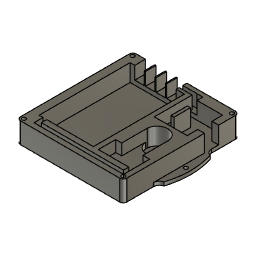
B07Z94FZSQ Wood Box v5 (Autodesk Fusion 360 design; units mm, degrees)
Autodesk Fusion 360 part; units mm, degrees
sketch "BoardDetails" plane through (0, 0, 0) normal (0, 0, 1) x (1, 0, 0)
  line L0 (6.7571, 3.9956, 17.5) -> (52.7571, 3.9956, 17.5)
  line L1 (52.7571, 3.9956, 17.5) -> (52.7571, 80.9956, 17.5)
  line L2 (52.7571, 80.9956, 17.5) -> (6.7571, 80.9956, 17.5)
  line L3 (6.7571, 80.9956, 17.5) -> (6.7571, 3.9956, 17.5)
  line L4 (29.7571, 80.9956, 17.5) -> (29.7571, 3.9956, 17.5) construction
  line L5 (29.7571, 80.9956, 17.5) -> (29.7571, 80.2494, 17.5)
  line L6 (29.7571, 80.9956, 17.5) -> (29.7571, 78.4956, 17.5) construction
  line L7 (29.7571, 78.4956, 17.5) -> (49.7571, 78.4956, 17.5) construction
  line L8 (29.7571, 78.4956, 17.5) -> (9.7571, 78.4956, 17.5) construction
  circle A0 through (12.0071, 78.4956, 17.5) (8.6321, 80.4442, 17.5) (8.6321, 76.5471, 17.5)
  circle A1 through (52.0071, 78.4956, 17.5) (48.6321, 80.4442, 17.5) (48.6321, 76.5471, 17.5)
  line L9 (29.7571, 3.9956, 17.5) -> (29.7571, 6.4956, 17.5)
  line L10 (29.7571, 6.4956, 17.5) -> (49.7571, 6.4956, 17.5) construction
  line L11 (29.7571, 6.4956, 17.5) -> (9.7571, 6.4956, 17.5) construction
  circle A2 through (12.0071, 6.4956, 17.5) (8.6321, 8.4442, 17.5) (8.6321, 4.5471, 17.5)
  circle A3 through (52.0071, 6.4956, 17.5) (48.6321, 8.4442, 17.5) (48.6321, 4.5471, 17.5)
  line L12 (62.0692, 18.5976, 17.5) -> (80.0692, 18.5976, 17.5)
  line L13 (80.0692, 18.5976, 17.5) -> (80.0692, 48.5976, 17.5)
  line L14 (80.0692, 48.5976, 17.5) -> (62.0692, 48.5976, 17.5)
  line L15 (62.0692, 48.5976, 17.5) -> (62.0692, 18.5976, 17.5)
  circle A4 through (80.095, 39.5718, 17.5) (66.5563, 47.3884, 17.5) (66.5563, 31.7552, 17.5)
  line L16 (85.7849, 18.5976, 17.5) -> (57.0002, 18.5976, 17.5)
  line L17 (57.0002, 18.5976, 17.5) -> (57.0002, 3.9337, 17.5)
  line L18 (57.0002, 3.9337, 17.5) -> (85.7849, 3.9337, 17.5)
  line L19 (85.7849, 3.9337, 17.5) -> (85.7849, 18.5976, 17.5)
  line L20 (84.3255, 51.6593, 17.5) -> (65.3255, 51.6593, 17.5)
  line L21 (65.3255, 51.6593, 17.5) -> (65.3255, 81.6593, 17.5)
  line L22 (65.3255, 81.6593, 17.5) -> (84.3255, 81.6593, 17.5)
  line L23 (84.3255, 81.6593, 17.5) -> (84.3255, 51.6593, 17.5)
  line L24 (84.3255, 66.6593, 17.5) -> (92.8255, 66.6593, 17.5)
  line L25 (92.8255, 72.6593, 17.5) -> (84.3255, 72.6593, 17.5)
  line L26 (84.3255, 72.6593, 17.5) -> (84.3255, 60.6593, 17.5)
  line L27 (84.3255, 60.6593, 17.5) -> (92.8255, 60.6593, 17.5)
  line L28 (92.8255, 60.6593, 17.5) -> (92.8255, 72.6593, 17.5)
  line L29 (92.8255, 72.6593, 17.5) -> (84.3255, 60.6593, 17.5) construction
  line L30 (84.3255, 72.6593, 17.5) -> (92.8255, 60.6593, 17.5) construction
  line L31 (65.3255, 51.6593, 17.5) -> (57.3255, 51.6593, 17.5)
  line L32 (57.3255, 51.6593, 17.5) -> (57.3255, 59.6593, 17.5)
  line L33 (57.3255, 59.6593, 17.5) -> (65.3255, 59.6593, 17.5)
  line L34 (65.3255, 59.6593, 17.5) -> (65.3255, 51.6593, 17.5)
  line L35 (65.3255, 81.6593, 17.5) -> (57.3255, 81.6593, 17.5)
  line L36 (57.3255, 81.6593, 17.5) -> (57.3255, 73.6593, 17.5)
  line L37 (57.3255, 73.6593, 17.5) -> (65.3255, 73.6593, 17.5)
  line L38 (65.3255, 73.6593, 17.5) -> (65.3255, 81.6593, 17.5)
  line L39 (85.8245, -0.5224, 17.5) -> (10.1189, -0.5224, 17.5)
  line L40 (10.1189, -0.5224, 17.5) -> (10.1189, -3.6224, 17.5)
  line L41 (10.1189, -3.6224, 17.5) -> (85.8245, -3.6224, 17.5)
  line L42 (85.8245, -3.6224, 17.5) -> (85.8245, -0.5224, 17.5)
  line L43 (10.1189, -0.5224, 17.5) -> (13.2189, -0.5224, 17.5)
  line L44 (13.2189, -0.5224, 17.5) -> (13.2189, 9.1628, 17.5)
  line L45 (13.2189, 9.1628, 17.5) -> (10.1189, 9.1628, 17.5)
  line L46 (10.1189, 9.1628, 17.5) -> (10.1189, -0.5224, 17.5)
  line L47 (85.8245, -0.5224, 17.5) -> (82.7245, -0.5224, 17.5)
  line L48 (82.7245, -0.5224, 17.5) -> (82.7245, 9.1628, 17.5)
  line L49 (82.7245, 9.1628, 17.5) -> (85.8245, 9.1628, 17.5)
  line L50 (85.8245, 9.1628, 17.5) -> (85.8245, -0.5224, 17.5)
  line L51 (6.7133, 80.7005, 17.5) -> (10.7133, 80.7005, 17.5)
  line L52 (10.7133, 80.7005, 17.5) -> (18.7133, 80.7005, 17.5)
  line L53 (18.7133, 80.7005, 17.5) -> (18.7133, 90.7005, 17.5)
  line L54 (18.7133, 90.7005, 17.5) -> (10.7133, 90.7005, 17.5)
  line L55 (10.7133, 90.7005, 17.5) -> (10.7133, 80.7005, 17.5)
  line L56 (18.7133, 80.7005, 17.5) -> (19.7133, 80.7005, 17.5)
  line L57 (19.7133, 80.7005, 17.5) -> (19.7133, 90.1133, 17.5)
  line L58 (19.7133, 90.1133, 17.5) -> (18.7133, 90.1133, 17.5)
  line L59 (18.7133, 90.1133, 17.5) -> (18.7133, 80.7005, 17.5)
  line L60 (19.7133, 80.7005, 17.5) -> (27.7133, 80.7005, 17.5)
  line L61 (27.7133, 80.7005, 17.5) -> (27.7133, 90.7005, 17.5)
  line L62 (27.7133, 90.7005, 17.5) -> (19.7133, 90.7005, 17.5)
  line L63 (19.7133, 90.7005, 17.5) -> (19.7133, 80.7005, 17.5)
  line L64 (27.7133, 80.7005, 17.5) -> (28.7133, 80.7005, 17.5)
  line L65 (28.7133, 80.7005, 17.5) -> (28.7133, 90.4026, 17.5)
  line L66 (28.7133, 90.4026, 17.5) -> (27.7133, 90.4026, 17.5)
  line L67 (27.7133, 90.4026, 17.5) -> (27.7133, 80.7005, 17.5)
  line L68 (28.7133, 80.7005, 17.5) -> (36.7133, 80.7005, 17.5)
  line L69 (36.7133, 80.7005, 17.5) -> (36.7133, 90.7005, 17.5)
  line L70 (36.7133, 90.7005, 17.5) -> (28.7133, 90.7005, 17.5)
  line L71 (28.7133, 90.7005, 17.5) -> (28.7133, 80.7005, 17.5)
  line L72 (36.7133, 80.7005, 17.5) -> (37.7133, 80.7005, 17.5)
  line L73 (37.7133, 80.7005, 17.5) -> (37.7133, 90.7005, 17.5)
  line L74 (37.7133, 90.7005, 17.5) -> (36.7133, 90.7005, 17.5)
  line L75 (36.7133, 90.7005, 17.5) -> (36.7133, 80.7005, 17.5)
  line L76 (37.7133, 80.7005, 17.5) -> (45.7133, 80.7005, 17.5)
  line L77 (45.7133, 80.7005, 17.5) -> (45.7133, 90.7005, 17.5)
  line L78 (45.7133, 90.7005, 17.5) -> (37.7133, 90.7005, 17.5)
  line L79 (37.7133, 90.7005, 17.5) -> (37.7133, 80.7005, 17.5)
  line L80 (45.7133, 83.4948, 17.5) -> (57.7133, 83.4948, 17.5)
  line L81 (57.7133, 83.4948, 17.5) -> (57.7133, 86.5948, 17.5)
  line L82 (57.7133, 86.5948, 17.5) -> (45.7133, 86.5948, 17.5)
  line L83 (45.7133, 86.5948, 17.5) -> (45.7133, 83.4948, 17.5)
  circle A5 centre (9.7649, 78.4891) radius 1
  circle A6 centre (49.8028, 78.4891) radius 1
  circle A7 centre (49.7195, 6.4968) radius 1.5
  circle A8 centre (9.7352, 6.4968) radius 1.5
  line L84 (62.7102, 86.5347, 17.5) -> (56.7102, 86.5347, 17.5)
  line L85 (56.7102, 86.5347, 17.5) -> (56.7102, 51.5347, 17.5)
  line L86 (56.7102, 51.5347, 17.5) -> (62.7102, 51.5347, 17.5)
  line L87 (62.7102, 51.5347, 17.5) -> (62.7102, 86.5347, 17.5)
  point P0 (84.3255, 66.6593)
  point P1 (88.5755, 66.6593)
  dimension "d3" = 46
  dimension "d4" = 77
  dimension "d5" = 2.5
  dimension "d6" = 20
  dimension "d7" = 20
  dimension "d8" = 4.5
  dimension "d9" = 4.5
  dimension "d10" = 2.5
  dimension "d11" = 20
  dimension "d12" = 20
  dimension "d13" = 4.5
  dimension "d14" = 4.5
  dimension "d18" = 18
  dimension "d19" = 30
  dimension "d20" = 19
  dimension "d21" = 30
  dimension "d24" = 12
  dimension "d35" = 3.1
  dimension "d36" = 3.1
  dimension "d37" = 3.1
  dimension "d40" = 4
  dimension "d41" = 8
  dimension "d42" = 10
  dimension "d43" = 1
  dimension "d44" = 8
  dimension "d45" = 10
  dimension "d46" = 1
  dimension "d47" = 8
  dimension "d48" = 10
  dimension "d49" = 1
  dimension "d50" = 10
  dimension "d51" = 8
  dimension "d52" = 10
  dimension "d53" = 12
  dimension "d54" = 3.1
  dimension "d59" = 2
  dimension "d60" = 2
  dimension "d61" = 3
  dimension "d62" = 3
  dimension "d65" = 6
  dimension "d66" = 35
  measures "d59" diameter of A5
  measures "d60" diameter of A6
  measures "d61" diameter of A7
  measures "d62" diameter of A8
sketch "WoodBoardDim" plane through (0, 0, 0) normal (0, 0, 1) x (1, 0, 0)
  line L0 (3, -8) -> (87, -8)
  line L1 (87, 90) -> (3, 90)
  line L2 (0, 17.5051) -> (0, -5)
  line L3 (0, -8) -> (0, 0)
  arc A0 (3, 90) -> (0, 87) centre (3, 87) ccw
  arc A1 (90, 87) -> (87, 90) centre (87, 87) ccw
  arc A2 (87, -8) -> (90, -5) centre (87, -5) ccw
  arc A3 (0, -5) -> (3, -8) centre (3, -5) ccw
  arc A4 (0, 17.5051) -> (-4, 22.4041) centre (-5, 17.5051) ccw
  line L4 (0, 66.4949) -> (0, 87)
  arc A5 (-4, 61.5959) -> (0, 66.4949) centre (-5, 66.4949) ccw
  line L5 (90, -5) -> (90, 17.5051)
  line L6 (90, 66.4949) -> (90, 87)
  arc A6 (90, 66.4949) -> (94, 61.5959) centre (95, 66.4949) ccw
  arc A7 (94, 22.4041) -> (90, 17.5051) centre (95, 17.5051) ccw
  line L7 (0, 66.4949) -> (0, 17.5051)
  line L8 (90, 17.5051) -> (90, 66.4949)
  circle A8 centre (3, 87) radius 1.6
  circle A9 centre (87, 87) radius 1.6
  circle A10 centre (3, -5) radius 1.6
  circle A11 centre (87, -5) radius 1.6
  circle A12 centre (-3, 42) radius 1.6
  circle A13 centre (93, 42) radius 1.6
  line L9 (-3, 42) -> (-7, 42)
  line L10 (93, 42) -> (97, 42)
  spline S0 degree 5 poles (-4, 61.5959) (-4.2275, 60.8121) (-4.6628, 59.2444) (-5.256, 56.8929) (-5.9257, 53.7576) (-6.5472, 49.8384) (-6.9337, 45.9192) (-7.066, 42) (-6.9337, 38.0808) (-6.5472, 34.1616) (-5.9257, 30.2424) (-5.256, 27.1071) (-4.6628, 24.7556) (-4.2275, 23.1879) (-4, 22.4041) knots 0 0 0 0 0 0 0.1 0.2 0.3 0.4 0.5 0.6 0.7 0.8 0.9 1 1 1 1 1 1
  spline S1 degree 5 poles (94, 61.5959) (94.2275, 60.8121) (94.6628, 59.2444) (95.256, 56.8929) (95.9257, 53.7576) (96.5472, 49.8384) (96.9337, 45.9192) (97.066, 42) (96.9337, 38.0808) (96.5472, 34.1616) (95.9257, 30.2424) (95.256, 27.1071) (94.6628, 24.7556) (94.2275, 23.1879) (94, 22.4041) knots 0 0 0 0 0 0 0.1 0.2 0.3 0.4 0.5 0.6 0.7 0.8 0.9 1 1 1 1 1 1
  dimension "d67" = 3
  dimension "d68" = 3
  dimension "d73" = 5
  dimension "d74" = 5
  dimension "d75" = 5
  dimension "d76" = 3.2
  dimension "d77" = 3.2
  dimension "d78" = 3.2
  dimension "d79" = 3.2
  dimension "d80" = 3.2
  dimension "d81" = 3.2
  dimension "d82" = 4
  dimension "d83" = 4
  constraint horizontal L0
  constraint vertical L5
  constraint horizontal L1
  constraint vertical L2
  constraint perpendicular L0 L3
  constraint tangent L2 A0
  constraint tangent L1 A0
  constraint tangent L1 A1
  constraint tangent A1 L5
  constraint tangent A2 L5
  constraint tangent L0 A2
  constraint equal A1 A2
  constraint coincident L0 L3.start
  constraint coincident L3.end L2
  constraint tangent L0 A3
  constraint tangent L2 A3
  constraint equal A1 A3
  constraint tangent L2 A4
  constraint tangent A0 L4
  constraint tangent L4 A5
  constraint collinear L5 L6
  constraint tangent L6 A6
  constraint tangent L5 A7
  constraint equal A6 A7
  constraint tangent A4 L7
  constraint concentric A0 A8
  constraint concentric A1 A9
  constraint concentric A3 A10
  constraint concentric A2 A11
  constraint coincident A12.centre L9.start
  constraint perpendicular L7 L9
  constraint coincident A13.centre L10.start
  constraint parallel L1 L10
  measures "d67" radius of A0
  measures "d68" radius of A1
  measures "d73" radius of A4
  measures "d74" radius of A5
  measures "d75" radius of A6
  measures "d76" diameter of A8
  measures "d77" diameter of A9
  measures "d78" diameter of A10
  measures "d79" diameter of A11
  measures "d80" diameter of A12
  measures "d81" diameter of A13
  measures "d82" distance of A12.centre L9.end
  measures "d83" distance of A13.centre L10.end
extrude "Extrude1" add sketch "WoodBoardDim" along normal blind 17.5 contours L0 L1 L2 L3 A0 A1 A2 A3 L4 L5 L6 L7 L8
extrude "Extrude2" cut sketch "BoardDetails" against normal blind 14.5 contours L0 L1 L2 L3 A0 A2 L44 L45 L46 L51 L52 L56 L60 L64 L68 L72 L76 L77 | L0 A2 L44 L45 L46 | L2 L73 L76 L77 L79 | A2 L46 | A2 L46 | L2 L69 L72 L73 L75 L79 | L2 L3 A0 L51 L55 | L2 L5 L68 L69 L75 | A0 L51 | A0 L51 | L2 L5 L65 L68 L71 | L2 L52 L53 L55 L59 | L2 L61 L64 L65 L67 L71 | L2 L53 L56 L57 L59 L63 | L2 L57 L60 L61 L63 L67 | L21 L31 L33 L34 L87 | L31 L32 L33 L87 | L13 L15 A4 | L35 L36 L37 L87 | L21 L35 L37 L38 L87 | L20 L21 L22 L23 L26 L34 L38 | L23 L24 L26 L27 L28 | L23 L24 L25 L26 L28 | A1 | A3 in plane through (0, 0, 17.5) normal (0, 0, 1)
extrude "Extrude3" cut sketch "BoardDetails" against normal blind 9.5 contours L18 L19 L48 L49 | L12 L16 L17 L18 L19 L48 L49 | L12 L13 L15 A4 L16 in plane through (0, 0, 17.5) normal (0, 0, 1)
extrude "Extrude4" cut sketch "BoardDetails" against normal blind 7.25 contours L0 L39 L43 L44 L46 | L0 A2 L44 L45 L46 | L39 L40 L41 L42 L43 L47 | L18 L19 L39 L47 L48 L49 L50 | L18 L19 L48 L49 in plane through (0, 0, 17.5) normal (0, 0, 1)
extrude "Extrude5" cut sketch "BoardDetails" against normal blind 10.875 contours L2 L73 L76 L77 L79 | L2 L73 L77 L78 L79 L83 | L77 L80 L81 L82 L83 L84 L85 | L2 L5 L68 L69 L75 | L2 L65 L69 L70 L71 L75 | L80 L81 L84 L85 | L31 L32 L33 L35 L36 L37 L80 L81 L84 L85 L86 L87 | L2 L5 L65 L68 L71 | L2 L53 L54 L55 L59 | L2 L52 L53 L55 L59 | L2 L57 L60 L61 L63 L67 | L2 L57 L61 L62 L63 L67 in plane through (0, 0, 17.5) normal (0, 0, 1)
extrude "Extrude7" add sketch "WoodBoardDim" along normal blind 3 contours A6 A7 L8 S1 | A4 A5 L7 S0
equation "WoodHeight = 17.5 mm"
equation "d16 = WoodHeight"
equation "BoxGround = 3 mm"
equation "WoodCarving = WoodHeight - BoxGround"
equation "d31 = -WoodCarving"
equation "d33 = -WoodCarving + 5 mm"
equation "d38 = -WoodCarving / 2"
equation "d57 = -WoodCarving * 0.75"
